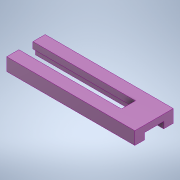
# Autodesk Inventor part: pistonHousingV03-8-in
Saved by Autodesk Inventor 2020.2 (Build 242310000, 310)
## iProperties
Created: 2020-01-19
Part Number: pistonHousingV03-8-in
Material: PET Plastic
Document SubType Name: Modeling
Designer: robst
Density: 1.541 g/cm^3
Appearance: Smooth - Purple
Author: robst
Autodesk Inventor part; units mm, degrees
ref_plane "YZ Plane" through (0, 0, 0) normal (1, 0, 0) x (0, 1, 0)
ref_plane "XZ Plane" through (0, 0, 0) normal (0, 1, 0) x (-1, 0, 0)
ref_plane "XY Plane" through (0, 0, 0) normal (0, 0, 1) x (1, 0, 0)
sketch "Sketch1" plane through (0, 0, 0) normal (0, 1, 0) x (-1, 0, 0)
  line L0 (127, 38.1) -> (-127, 38.1)
  line L1 (-127, 38.1) -> (-127, -38.1)
  line L2 (-127, -38.1) -> (127, -38.1)
  line L3 (127, -38.1) -> (127, 38.1)
  line L4 (127, 38.1) -> (-127, -38.1) construction
  line L5 (-127, 38.1) -> (127, -38.1) construction
  point P0 (0, 0)
  dimension "d0" = 254
  dimension "d1" = 76.2
  constraints: 12 end point, 2 midpoint, 2 parallel, 1 horizontal, 1 perpendicular
  measures "d0" distance of L0.start L0.end
  measures "d1" distance of L1.end L0.end
extrude "Extrusion1" add sketch "Sketch1" along normal blind 25.4
sketch "Sketch2" plane through (0, 0, 0) normal (0, -1, 0) x (1, 0, 0)
  line L0 (-127, 19.05) -> (-127, -19.05)
  line L1 (-127, -19.05) -> (127, -19.05)
  line L2 (127, -19.05) -> (127, 19.05)
  line L3 (127, 19.05) -> (-127, 19.05)
  line L4 (-127, 19.05) -> (127, -19.05) construction
  line L5 (-127, -19.05) -> (127, 19.05) construction
  point P0 (0, 0)
  dimension "d4" = 38.1
  constraints: 12 end point, 2 midpoint, 2 parallel, 1 perpendicular, 1 vertical
  measures "d4" distance of L0.start L0.end
extrude "Extrusion2" cut sketch "Sketch2" against normal blind 12.7
sketch "Sketch3" plane through (0, 12.7, 0) normal (0, -1, 0) x (1, 0, 0)
  line L0 (-127, -19.05) -> (-127, 19.05) projected
  line L1 (76.2, 13.97) -> (76.2, -13.97)
  line L2 (76.2, -13.97) -> (-127, -13.97)
  line L3 (-127, -13.97) -> (-127, 13.97)
  line L4 (-127, 13.97) -> (76.2, 13.97)
  line L5 (76.2, 13.97) -> (-127, -13.97) construction
  line L6 (76.2, -13.97) -> (-127, 13.97) construction
  point P0 (0, 0)
  point P1 (-25.4, 0)
  point P2 (-127, -13.97)
  dimension "d7" = 101.6
  dimension "d8" = 27.94
  constraints: 12 end point, 2 midpoint, 2 parallel, 1 perpendicular, 1 vertical
  measures "d7" distance from line of point (-25.4, 0) L0
  measures "d8" distance of L1.start L1.end
extrude "Extrusion3" cut sketch "Sketch3" against normal through all
body "Solid1"
